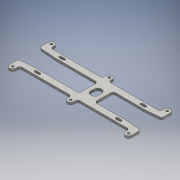
# Autodesk Inventor part: updown_slider
Saved by Autodesk Inventor 2016 (Build 200138000, 138)
## iProperties
Created: 2015-12-08
Part Number: updown_slider
Material: Generic
Document SubType Name: Modeling
Designer: lk8187
Density: 1 g/cm^3
Appearance: Smooth - Light Gray
Author: lk8187
Autodesk Inventor part; units mm, degrees
ref_plane "YZ Plane" through (0, 0, 0) normal (1, 0, 0) x (0, 1, 0)
ref_plane "XZ Plane" through (0, 0, 0) normal (0, 1, 0) x (-1, 0, 0)
ref_plane "XY Plane" through (0, 0, 0) normal (0, 0, 1) x (1, 0, 0)
sketch "Sketch1" plane through (0, 0, 0) normal (0, 0, 1) x (1, 0, 0)
  line L0 (135.5, -53.5) -> (140.5, -53.5)
  arc A0 (140.5, -56.5) -> (140.5, -53.5) centre (140.5, -55) ccw
  line L1 (140.5, -56.5) -> (135.5, -56.5)
  arc A1 (135.5, -53.5) -> (135.5, -56.5) centre (135.5, -55) ccw
  line L2 (30.5, -21.5) -> (35.5, -21.5)
  arc A2 (35.5, -24.5) -> (35.5, -21.5) centre (35.5, -23) ccw
  line L3 (35.5, -24.5) -> (30.5, -24.5)
  arc A3 (30.5, -21.5) -> (30.5, -24.5) centre (30.5, -23) ccw
  line L4 (35.5, -56.5) -> (30.5, -56.5)
  arc A4 (30.5, -53.5) -> (30.5, -56.5) centre (30.5, -55) ccw
  line L5 (30.5, -53.5) -> (35.5, -53.5)
  arc A5 (35.5, -56.5) -> (35.5, -53.5) centre (35.5, -55) ccw
  line L6 (140.5, -24.5) -> (135.5, -24.5)
  arc A6 (135.5, -21.5) -> (135.5, -24.5) centre (135.5, -23) ccw
  line L7 (135.5, -21.5) -> (140.5, -21.5)
  arc A7 (140.5, -24.5) -> (140.5, -21.5) centre (140.5, -23) ccw
  arc A8 (6.0006, -22.6082) -> (8.7763, -25.5998) centre (9.0006, -22.6082) ccw
  line L8 (8.7763, -25.5998) -> (27.4457, -27)
  arc A9 (27.2213, -26.9916) -> (27.4457, -27) centre (27.4457, -24) ccw
  line L9 (27.4457, -27) -> (80, -27)
  arc A10 (83, -30) -> (80, -27) centre (80, -30) ccw
  line L10 (83, -30) -> (83, -48.0084)
  arc A11 (80, -51.0084) -> (83, -48.0084) centre (80, -48.0084) ccw
  line L11 (80, -51.0084) -> (27.2213, -51.0084)
  arc A12 (27.4457, -51) -> (27.2213, -51.0084) centre (27.4457, -54) ccw
  line L12 (27.2213, -51.0084) -> (8.7756, -52.3918)
  arc A13 (8.7756, -52.3918) -> (6, -55.3834) centre (9, -55.3834) ccw
  line L13 (6, -55.3834) -> (6, -64)
  arc A14 (6, -64) -> (14, -64) centre (10, -64) ccw
  line L14 (14, -64) -> (14, -62)
  arc A15 (17, -59) -> (14, -62) centre (17, -62) ccw
  line L15 (17, -59) -> (78, -59)
  arc A16 (81, -62) -> (78, -59) centre (78, -62) ccw
  line L16 (81, -62) -> (81, -64)
  arc A17 (81, -64) -> (89, -64) centre (85, -64) ccw
  line L17 (89, -64) -> (89, -62)
  arc A18 (92, -59) -> (89, -62) centre (92, -62) ccw
  line L18 (92, -59) -> (152.9994, -59)
  arc A19 (155.9994, -62) -> (152.9994, -59) centre (152.9994, -62) ccw
  line L19 (155.9994, -62) -> (155.9994, -64)
  arc A20 (155.9994, -64) -> (163.9994, -64) centre (159.9994, -64) ccw
  line L20 (163.9994, -64) -> (163.9994, -55.3918)
  arc A21 (163.9994, -55.3918) -> (161.2237, -52.4002) centre (160.9994, -55.3918) ccw
  line L21 (161.2237, -52.4002) -> (142.5543, -51)
  arc A22 (142.7787, -51.0084) -> (142.5543, -51) centre (142.5543, -54) ccw
  line L22 (142.5543, -51) -> (106, -51)
  arc A23 (103, -48) -> (106, -51) centre (106, -48) ccw
  line L23 (103, -48) -> (103, -29.9916)
  arc A24 (106, -26.9916) -> (103, -29.9916) centre (106, -29.9916) ccw
  line L24 (106, -26.9916) -> (142.7787, -26.9916)
  arc A25 (142.5543, -27) -> (142.7787, -26.9916) centre (142.5543, -24) ccw
  line L25 (142.7787, -26.9916) -> (161.2244, -25.6082)
  arc A26 (161.2244, -25.6082) -> (164.0006, -22.6166) centre (161.0006, -22.6165) ccw
  line L26 (164.0006, -22.6166) -> (164.0006, -14)
  arc A27 (164.0006, -14) -> (156.0006, -14) centre (160.0006, -14) ccw
  line L27 (156.0006, -14) -> (156.0006, -16)
  arc A28 (153.0006, -19) -> (156.0006, -16) centre (153.0006, -16) ccw
  line L28 (153.0006, -19) -> (92.0006, -19)
  arc A29 (89.0006, -16) -> (92.0006, -19) centre (92.0006, -16) ccw
  line L29 (89.0006, -16) -> (89.0006, -14)
  arc A30 (89.0006, -14) -> (81.0006, -14) centre (85.0006, -14) ccw
  line L30 (81.0006, -14) -> (81.0006, -16)
  arc A31 (78.0006, -19) -> (81.0006, -16) centre (78.0006, -16) ccw
  line L31 (78.0006, -19) -> (17.0006, -19)
  arc A32 (14.0006, -16) -> (17.0006, -19) centre (17.0006, -16) ccw
  line L32 (14.0006, -16) -> (14.0006, -14)
  arc A33 (14.0006, -14) -> (6.0006, -14) centre (10.0006, -14) ccw
  line L33 (6.0006, -14) -> (6.0006, -22.6082)
  arc A34 (98, -37) -> (88, -37) centre (93, -37) ccw
  line L34 (98, -37) -> (98, -41)
  arc A35 (88, -41) -> (98, -41) centre (93, -41) ccw
  line L35 (88, -41) -> (88, -37)
  circle A36 centre (10, -14) radius 1.5
  circle A37 centre (10, -64) radius 1.5
  circle A38 centre (85, -64) radius 1.5
  circle A39 centre (85, -14) radius 1.5
  circle A40 centre (160, -14) radius 1.5
  circle A41 centre (160, -64) radius 1.5
  point P0 (0, 0)
  constraints: 72 end point, 72 point on circle, 42 centre point
extrude "Extrusion1" add sketch "Sketch1" along normal blind 3
body "Solid1"
